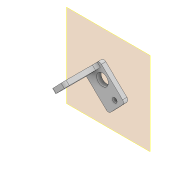
# Autodesk Inventor part: IM_Lensholder_motorized
Saved by Autodesk Inventor 2022 (Build 260153000, 153)
## iProperties
Created: 2023-08-15
Part Number: IM_Lensholder_motorized
Material: Generisch
Document SubType Name: Modeling
Designer: diederichbenedict
Density: 1 g/cm^3
Appearance: Vorgabe
Author: diederichbenedict
Autodesk Inventor part; units mm, degrees
ref_plane "YZ Plane" through (0, 0, 0) normal (1, 0, 0) x (0, 1, 0)
ref_plane "XZ Plane" through (0, 0, 0) normal (0, 1, 0) x (-1, 0, 0)
ref_plane "Arbeitsebene3" through (94.1454, 44.3915, -66.8179) normal (0, 0, 1) x (1, 0.0000007, 0)
sketch "Skizze4" plane through (94.1454, 44.3915, -66.8179) normal (0, 0, 1) x (1, 0.0000007, 0)
  circle A0 centre (0.0001, -0.0022) radius 3.9802
  circle A1 centre (8.3745, -8.0022) radius 1.4
  line L0 (-5.8906, 8.1313) -> (-10.0357, 3.7933)
  line L1 (-9.5056, 11.5855) -> (-5.8906, 8.1313)
  line L2 (-10.0357, 3.7933) -> (-10.7515, 3.0441)
  line L3 (-10.7515, 3.0441) -> (-13.0827, 0.6044)
  line L4 (-5.8906, 8.1313) -> (-1.3114, 3.7557)
  line L5 (2.9045, 2.7193) -> (12.9558, -6.8851)
  line L6 (12.9558, -6.8851) -> (3.1712, -17.1251)
  line L7 (3.1712, -17.1251) -> (-14.1808, -0.5447)
  line L8 (-14.1808, -0.5447) -> (-13.0914, 0.5954)
  line L9 (-16.6977, 4.0587) -> (-13.0827, 0.6044)
  line L10 (-17.7958, 2.9095) -> (-16.6977, 4.0587)
  line L11 (-17.7958, 2.9095) -> (-14.1808, -0.5447)
  line L12 (-13.0827, 0.6044) -> (-14.1808, -0.5447)
  line L13 (12.9558, -6.8851) -> (14.2248, -5.5571)
  line L14 (14.2248, -5.5571) -> (-3.1272, 11.0232)
  line L15 (-3.1272, 11.0232) -> (-5.8906, 8.1313)
  line L16 (-37.4679, 35.8018) -> (37.4679, -35.8018)
  circle A2 centre (-0.9396, 0.8978) radius 4
  circle A3 centre (7.4327, -7.1022) radius 1.6
  point P0 (-94.1455, -44.3914)
extrude "Extrusion4" add sketch "Skizze4" along normal blind 3 contours A0 L16 A2 | A0 L5 L6 L16 A1 A3 | A0 A2 L4 L15 L14 L13 L5 | L16 A3 A1 L6 L7 L8 L12 L3 L2 L0 A2 A0 | A0 A2 L16 | A2 L16 L0 L4 | A1 L16 A3 | A3 L16 A1 picked at (2.5745, -1.7629) picked at (2.3182, -2.6617) picked at (8.9731, -8.3119) picked at (8.6694, -8.6141)
sketch "Skizze5" plane through (94.1454, 44.3915, -63.8179) normal (0, 0, 1) x (1, 0.0000007, 0)
  line L0 (-16.6977, 4.0587) -> (-13.0827, 0.6044) projected
  line L1 (-17.7958, 2.9095) -> (-16.6977, 4.0587) projected
  line L2 (-17.7958, 2.9095) -> (-14.1808, -0.5447) projected
  line L3 (-13.0827, 0.6044) -> (-14.1808, -0.5447) projected
  line L4 (-9.5056, 11.5855) -> (-5.8906, 8.1313) projected
  line L5 (14.2248, -5.5571) -> (-3.1272, 11.0232) projected
  line L6 (-3.1272, 11.0232) -> (-14.1808, -0.5447) projected
  line L7 (-14.1808, -0.5447) -> (3.1712, -17.1251) projected
  line L8 (3.1712, -17.1251) -> (14.2248, -5.5571) projected
  line L9 (-3.1272, 11.0232) -> (-14.1808, -0.5447) projected
  line L10 (-14.1808, -0.5447) -> (-5.8906, 8.1313)
  line L11 (-5.8906, 8.1313) -> (-3.7216, 6.0587)
  line L12 (-3.7216, 6.0587) -> (-12.0118, -2.6173)
  line L13 (-12.0118, -2.6173) -> (-14.1808, -0.5447)
  point P0 (-94.1455, -44.3914)
  point P1 (-12.0118, -2.6173)
  point P2 (-5.8906, 8.1313)
  point P3 (-13.0827, 0.6044)
  point P4 (-14.1808, -0.5447)
  dimension "d20" = 3
  constraints: 8 end point, 2 parallel, 1 collinear, 1 perpendicular
  measures "d20" distance of L4.end L11.end
ref_plane "Arbeitsebene4" through (80.4947, 48.1847, -41.8179) normal (0, 0, 1) x (0.722999, -0.6908491, 0)
extrude "Extrusion5" add sketch "Skizze5" along normal up to surface (22 mm away) contours L6 L11 L12 L7 L3
sketch "Skizze6" plane through (82.1336, 41.7742, -41.8179) normal (0.722999, -0.6908491, 0) x (0, 0, -1)
  circle A0 centre (2, 10.1654) radius 0.5 projected
  circle A1 centre (2, 3.5654) radius 0.5 projected
  point P0 (-41.8179, -86.9446)
extrude "Extrusion6" cut sketch "Skizze6" against normal blind 10
fillet "Rundung1" radius 2 6 edges at (81.0491, 42.8105, -41.8179) (89.3393, 51.4865, -41.8179) (97.3166, 27.2664, -65.3179) (108.3702, 38.8343, -65.3179) (89.3393, 51.4865, -63.8179) (91.0182, 55.4147, -65.3179)
